Autodesk Fusion 360 part; units mm, degrees
(part 2 of 2)
sketch "Sketch4" plane through (0, 0, 5) normal (0, 0, 1) x (-1, 0, 0)
  circle A0 centre (-30, 34) radius 1.15
  circle A1 centre (-30, 82) radius 1.4
  circle A2 centre (27, 86) radius 1.15
  circle A3 centre (35, 78) radius 1.15
  circle A4 centre (31, 34) radius 1.4
  circle A5 centre (-81, 66.5) radius 1.15
  circle A6 centre (-89, 26.5) radius 1.15
  circle A7 centre (-45, 26.5) radius 1.4
  circle A8 centre (-45, 8) radius 1.15
  circle A9 centre (46, 26.5) radius 1.15
  circle A10 centre (90.029, 26.5184) radius 1.4
  circle A11 centre (90, 8) radius 1.15
  circle A12 centre (-85, 16) radius 1.15
  circle A13 centre (-85.0037, -28) radius 1.4
  circle A14 centre (-45, -32) radius 1.15
  circle A15 centre (50, -24) radius 1.15
  circle A16 centre (49.9963, -28) radius 1.4
  circle A17 centre (50, 16) radius 1.15
  circle A18 centre (-85, -32) radius 1.15
  circle A19 centre (-85, 12) radius 1.4
  circle A20 centre (90, -24) radius 1.15
  circle A21 centre (94.029, 26.5184) radius 1.15
  circle A22 centre (50, 26.5) radius 1.4
  circle A23 centre (94, 66.5) radius 1.15
  circle A24 centre (-41, 26.5) radius 1.15
  circle A25 centre (-85, 26.5) radius 1.4
  circle A26 centre (-85, 56) radius 1.15
  circle A27 centre (35, 34) radius 1.15
  circle A28 centre (35, 42) radius 1.15
  circle A29 centre (31, 86) radius 1.4
  circle A30 centre (-30, 86) radius 1.15
  circle A31 centre (-26, 34) radius 1.4
  circle A32 centre (-30, 38) radius 1.4
  circle A33 centre (-30, 78) radius 1.15
  circle A34 centre (-22, 86) radius 1.15
  circle A35 centre (35, 82) radius 1.4
  circle A36 centre (27, 34) radius 1.15
  circle A37 centre (-85, 66.5) radius 1.4
  circle A38 centre (-85, 48) radius 1.15
  circle A39 centre (-49, 26.5) radius 1.15
  circle A40 centre (-45, 12) radius 1.4
  circle A41 centre (86, 66.5) radius 1.15
  circle A42 centre (86.029, 26.5184) radius 1.15
  circle A43 centre (90, 12) radius 1.4
  circle A44 centre (90, -32) radius 1.15
  circle A45 centre (-85, -24) radius 1.15
  circle A46 centre (-45.0037, -28) radius 1.4
  circle A47 centre (50, 8) radius 1.15
  circle A48 centre (50, -32) radius 1.15
  circle A49 centre (50, 12) radius 1.4
  circle A50 centre (-45, -24) radius 1.15
  circle A51 centre (-85, 8) radius 1.15
  circle A52 centre (89.9963, -28) radius 1.4
  circle A53 centre (90, 16) radius 1.15
  circle A54 centre (54, 26.5) radius 1.15
  circle A55 centre (90, 66.5) radius 1.4
  circle A56 centre (-45, 16) radius 1.15
  circle A57 centre (-81, 26.5) radius 1.15
  circle A58 centre (-85, 52) radius 1.4
  circle A59 centre (-89, 66.5) radius 1.15
  circle A60 centre (35, 38) radius 1.4
  circle A61 centre (35, 86) radius 1.15
  circle A62 centre (-26, 86) radius 1.4
  circle A63 centre (-22, 34) radius 1.15
  circle A64 centre (-30, 42) radius 1.15
  circle A65 centre (65.5, 46) radius 2
  arc A66 (-39.1, -77.6) -> (-39.1, -74.4) centre (-39.1, -76) ccw
  line L0 (-39.1, -77.6) -> (-46.9, -77.6)
  arc A67 (-46.9, -74.4) -> (-46.9, -77.6) centre (-46.9, -76) ccw
  line L1 (-46.9, -74.4) -> (-39.1, -74.4)
  circle A68 centre (75.5, -43.5) radius 1.35
  arc A69 (-53.1, -93.6) -> (-53.1, -90.4) centre (-53.1, -92) ccw
  line L2 (-53.1, -93.6) -> (-60.9, -93.6)
  arc A70 (-60.9, -90.4) -> (-60.9, -93.6) centre (-60.9, -92) ccw
  line L3 (-60.9, -90.4) -> (-53.1, -90.4)
  arc A71 (65.9, -93.6) -> (65.9, -90.4) centre (65.9, -92) ccw
  line L4 (65.9, -93.6) -> (58.1, -93.6)
  arc A72 (58.1, -90.4) -> (58.1, -93.6) centre (58.1, -92) ccw
  line L5 (58.1, -90.4) -> (65.9, -90.4)
  circle A73 centre (-62.5, -48.623) radius 1.15
  arc A74 (51.9, -77.6) -> (51.9, -74.4) centre (51.9, -76) ccw
  line L6 (51.9, -77.6) -> (44.1, -77.6)
  arc A75 (44.1, -74.4) -> (44.1, -77.6) centre (44.1, -76) ccw
  line L7 (44.1, -74.4) -> (51.9, -74.4)
  arc A76 (90.4506, 78.0996) -> (95.5506, 78.099) centre (93.0006, 78.099) ccw
  line L8 (90.4506, 78.0996) -> (90.4506, 84.449)
  line L9 (90.4506, 84.449) -> (84.1006, 84.449)
  arc A77 (84.1006, 89.549) -> (84.1006, 84.449) centre (84.1006, 86.999) ccw
  line L10 (84.1006, 89.549) -> (92.9866, 89.549)
  arc A78 (94.8063, 88.7996) -> (92.9866, 89.549) centre (93.0006, 86.9991) ccw
  arc A79 (95.5506, 86.985) -> (94.8063, 88.7996) centre (93.0006, 86.999) ccw
  line L11 (95.5506, 86.985) -> (95.5506, 78.099)
  circle A80 centre (67.5, -48.623) radius 1.15
  arc A81 (51.9, -93.6) -> (51.9, -90.4) centre (51.9, -92) ccw
  line L12 (51.9, -93.6) -> (44.1, -93.6)
  arc A82 (44.1, -90.4) -> (44.1, -93.6) centre (44.1, -92) ccw
  line L13 (44.1, -90.4) -> (51.9, -90.4)
  arc A83 (65.9, -77.6) -> (65.9, -74.4) centre (65.9, -76) ccw
  line L14 (65.9, -77.6) -> (58.1, -77.6)
  arc A84 (58.1, -74.4) -> (58.1, -77.6) centre (58.1, -76) ccw
  line L15 (58.1, -74.4) -> (65.9, -74.4)
  circle A85 centre (-60.5, 85) radius 2
  arc A86 (-23, -94.551) -> (-22.9994, -89.451) centre (-22.9994, -92.001) ccw
  line L16 (-23, -94.551) -> (-31.8994, -94.551)
  arc A87 (-31.8994, -89.451) -> (-31.8994, -94.551) centre (-31.8994, -92.001) ccw
  line L17 (-31.8994, -89.451) -> (-22.9994, -89.451)
  circle A88 centre (-81.5, -43.5) radius 1.35
  circle A89 centre (65.5, 85) radius 2
  circle A90 centre (65.5, 65.5) radius 15
  arc A91 (36.9, -94.551) -> (36.9006, -89.451) centre (36.9006, -92.001) ccw
  line L18 (36.9, -94.551) -> (28.0006, -94.551)
  arc A92 (28.0006, -89.451) -> (28.0006, -94.551) centre (28.0006, -92.001) ccw
  line L19 (28.0006, -89.451) -> (36.9006, -89.451)
  arc A93 (-79, 84.449) -> (-78.9994, 89.549) centre (-78.9994, 86.999) ccw
  line L20 (-79, 84.449) -> (-85.3494, 84.449)
  line L21 (-85.3494, 84.449) -> (-85.3494, 78.099)
  arc A94 (-90.4494, 78.099) -> (-85.3494, 78.099) centre (-87.8994, 78.099) ccw
  line L22 (-90.4494, 78.099) -> (-90.4494, 86.9852)
  arc A95 (-89.7213, 88.7832) -> (-90.4494, 86.9852) centre (-87.8994, 86.999) ccw
  arc A96 (-87.8854, 89.549) -> (-89.7213, 88.7832) centre (-87.8994, 86.9991) ccw
  line L23 (-87.8854, 89.549) -> (-78.9994, 89.549)
  arc A97 (37.9, -77.6) -> (37.9, -74.4) centre (37.9, -76) ccw
  line L24 (37.9, -77.6) -> (30.1, -77.6)
  arc A98 (30.1, -74.4) -> (30.1, -77.6) centre (30.1, -76) ccw
  line L25 (30.1, -74.4) -> (37.9, -74.4)
  circle A99 centre (-60.5, 65.5) radius 15
  circle A100 centre (67.5, -59.5) radius 1.15
  circle A101 centre (-70.5, -43.5) radius 1.35
  arc A102 (-53.1, -77.6) -> (-53.1, -74.4) centre (-53.1, -76) ccw
  line L26 (-53.1, -77.6) -> (-60.9, -77.6)
  arc A103 (-60.9, -74.4) -> (-60.9, -77.6) centre (-60.9, -76) ccw
  line L27 (-60.9, -74.4) -> (-53.1, -74.4)
  circle A104 centre (-92.5, -43.5) radius 1.35
  arc A105 (-25.1, -77.6) -> (-25.1, -74.4) centre (-25.1, -76) ccw
  line L28 (-25.1, -77.6) -> (-32.9, -77.6)
  arc A106 (-32.9, -74.4) -> (-32.9, -77.6) centre (-32.9, -76) ccw
  line L29 (-32.9, -74.4) -> (-25.1, -74.4)
  circle A107 centre (86.5, -43.5) radius 1.35
  circle A108 centre (-62.5, -59.5) radius 1.15
  circle A109 centre (-60.5, 46) radius 2
  circle A110 centre (97.5, -43.5) radius 1.35
  arc A111 (-39.1, -93.6) -> (-39.1, -90.4) centre (-39.1, -92) ccw
  line L30 (-39.1, -93.6) -> (-46.9, -93.6)
  arc A112 (-46.9, -90.4) -> (-46.9, -93.6) centre (-46.9, -92) ccw
  line L31 (-46.9, -90.4) -> (-39.1, -90.4)
  line L32 (-67.5, -102.5) -> (72.5, -102.5)
  line L33 (72.5, -102.5) -> (72.5, -47.5)
  line L34 (72.5, -47.5) -> (102.5, -47.5)
  line L35 (102.5, -47.5) -> (102.5, 97.5)
  line L36 (102.5, 97.5) -> (-97.5, 97.5)
  line L37 (-97.5, 97.5) -> (-97.5, -47.5)
  line L38 (-97.5, -47.5) -> (-67.5, -47.5)
  line L39 (-67.5, -47.5) -> (-67.5, -102.5)
  circle A113 centre (2.5, 10) radius 1.15
  circle A114 centre (2.5, 2) radius 1.15
  circle A115 centre (-26.5, -23) radius 1.4
  circle A116 centre (23.5, -19) radius 1.15
  circle A117 centre (31.5, -19) radius 1.15
  circle A118 centre (2.5, -44) radius 1.4
  circle A119 centre (6.5, -48) radius 1.4
  circle A120 centre (10.5, -48) radius 1.15
  circle A121 centre (-5.5, -48) radius 1.15
  circle A122 centre (31.5, -23) radius 1.4
  circle A123 centre (27.5, -19) radius 1.4
  circle A124 centre (-26.5, -19) radius 1.15
  circle A125 centre (-26.5, -11) radius 1.15
  circle A126 centre (10.5, 10) radius 1.15
  circle A127 centre (-1.5, 10) radius 1.4
  circle A128 centre (2.5, 6) radius 1.4
  circle A129 centre (-26.5, -27) radius 1.15
  circle A130 centre (-18.5, -19) radius 1.15
  circle A131 centre (31.5, -15) radius 1.4
  circle A132 centre (2.5, -40) radius 1.15
  circle A133 centre (2.5, -48) radius 1.15
  circle A134 centre (-1.5, -48) radius 1.4
  circle A135 centre (31.5, -27) radius 1.15
  circle A136 centre (31.5, -11) radius 1.15
  circle A137 centre (-22.5, -19) radius 1.4
  circle A138 centre (-26.5, -15) radius 1.4
  circle A139 centre (6.5, 10) radius 1.4
  circle A140 centre (-5.5, 10) radius 1.15
  circle A141 centre (62.5, -100) radius 1.15
  circle A142 centre (-27.5, -100) radius 1.15
  circle A143 centre (47.5, -100) radius 1.15
  circle A144 centre (-57.5, -100) radius 1.15
  circle A145 centre (-42.5, -100) radius 1.15
  circle A146 centre (32.5, -100) radius 1.15
sketch "Sketch5" plane through (0, 0, 8) normal (0, 0, 1) x (-1, 0, 0)
  circle A0 centre (90.029, 26.5184) radius 1.4
  circle A1 centre (-45, 12) radius 1.4
  circle A2 centre (86, 66.5) radius 1.15
  circle A3 centre (-45, -32) radius 1.15
  circle A4 centre (50, -32) radius 1.15
  circle A5 centre (90, 66.5) radius 1.4
  circle A6 centre (-89, 26.5) radius 1.15
  circle A7 centre (-45.0037, -28) radius 1.4
  line L0 (-42, 23.5) -> (47, 23.5)
  line L1 (47, 23.5) -> (47, 15.996)
  line L2 (47, 15.996) -> (47.0104, 8.2491)
  arc A8 (47.0104, 8.2491) -> (47, 7.9983) centre (50, 8) ccw
  line L3 (47, 7.9983) -> (47, -24.0028)
  line L4 (47, -24.0028) -> (47.0072, -31.7917)
  arc A9 (47.0072, -31.7917) -> (47, -31.9983) centre (50, -32) ccw
  line L5 (47, -31.9983) -> (47, -61.5)
  line L6 (47, -61.5) -> (-42, -61.5)
  line L7 (-42, -61.5) -> (-42, 23.5)
  circle A10 centre (54, 26.5) radius 1.15
  circle A11 centre (49.9963, -28) radius 1.4
  circle A12 centre (-45, 8) radius 1.15
  circle A13 centre (-45, 16) radius 1.15
  circle A14 centre (-85, 66.5) radius 1.4
  circle A15 centre (-45, -24) radius 1.15
  circle A16 centre (50, -24) radius 1.15
  circle A17 centre (50, 16) radius 1.15
  circle A18 centre (50, 12) radius 1.4
  circle A19 centre (-81, 66.5) radius 1.15
  circle A20 centre (86.029, 26.5184) radius 1.15
  circle A21 centre (50, 26.5) radius 1.4
  circle A22 centre (50, 8) radius 1.15
  circle A23 centre (46, 26.5) radius 1.15
  circle A24 centre (-45, 26.5) radius 1.4
  circle A25 centre (-81, 26.5) radius 1.15
  circle A26 centre (94.029, 26.5184) radius 1.15
  circle A27 centre (-49, 26.5) radius 1.15
  circle A28 centre (-41, 26.5) radius 1.15
  circle A29 centre (-85, 26.5) radius 1.4
  circle A30 centre (-89, 66.5) radius 1.15
  circle A31 centre (94, 66.5) radius 1.15
  line L8 (-92.5, -40.1151) -> (-89.5, -40.1151)
  line L9 (-89.5, -40.1151) -> (-89.5, 23.542)
  arc A32 (-89.5, 23.542) -> (-88.996, 23.5) centre (-89, 26.5) ccw
  line L10 (-88.996, 23.5) -> (-81.2491, 23.5104)
  arc A33 (-81.2491, 23.5104) -> (-81.0018, 23.5) centre (-81, 26.5) ccw
  line L11 (-81.0018, 23.5) -> (-48, 23.5)
  line L12 (-48, 23.5) -> (-48, 15.996)
  line L13 (-48, 15.996) -> (-47.9896, 8.2491)
  arc A34 (-47.9896, 8.2491) -> (-48, 7.9983) centre (-45, 8) ccw
  line L14 (-48, 7.9983) -> (-48, -24.0028)
  line L15 (-48, -24.0028) -> (-47.9928, -31.7917)
  arc A35 (-47.9928, -31.7917) -> (-48, -32.0017) centre (-45, -32) ccw
  line L16 (-48, -32.0017) -> (-48, -61.5)
  line L17 (-48, -61.5) -> (-59, -61.5)
  line L18 (-59, -61.5) -> (-59, -67.5)
  line L19 (-59, -67.5) -> (-67.5, -67.5)
  line L20 (-67.5, -67.5) -> (-67.5, -70.5)
  line L21 (-67.5, -70.5) -> (-17.5, -70.5)
  line L22 (-17.5, -70.5) -> (-17.5, -97.5)
  line L23 (-17.5, -97.5) -> (-67.5, -97.5)
  line L24 (-67.5, -97.5) -> (-67.5, -102.5)
  line L25 (-67.5, -102.5) -> (-15, -102.5)
  line L26 (-15, -102.5) -> (-15, -67.5)
  line L27 (-15, -67.5) -> (20, -67.5)
  line L28 (20, -67.5) -> (20, -102.5)
  line L29 (20, -102.5) -> (72.5, -102.5)
  line L30 (72.5, -102.5) -> (72.5, -97.5)
  line L31 (72.5, -97.5) -> (22.5, -97.5)
  line L32 (22.5, -97.5) -> (22.5, -70.5)
  line L33 (22.5, -70.5) -> (72.5, -70.5)
  line L34 (72.5, -70.5) -> (72.5, -67.5)
  line L35 (72.5, -67.5) -> (64, -67.5)
  line L36 (64, -67.5) -> (64, -61.5)
  line L37 (64, -61.5) -> (53, -61.5)
  line L38 (53, -61.5) -> (53, 23.5)
  line L39 (53, 23.5) -> (94.5, 23.5)
  line L40 (94.5, 23.5) -> (94.5, -40.1151)
  line L41 (94.5, -40.1151) -> (97.5, -40.1151)
  line L42 (97.5, -40.1151) -> (97.5, 69.5047)
  line L43 (97.5, 69.5047) -> (86.2491, 69.4896)
  arc A36 (86.2491, 69.4896) -> (86, 63.5) centre (86, 66.5) ccw
  line L44 (86, 63.5) -> (94, 63.5)
  line L45 (94, 63.5) -> (94.5, 63.5)
  line L46 (94.5, 63.5) -> (94.5, 29.4812)
  arc A37 (94.5, 29.4812) -> (94.361, 29.5) centre (94.029, 26.5184) ccw
  line L47 (94.361, 29.5) -> (59, 29.5)
  line L48 (59, 29.5) -> (47, 41.5)
  line L49 (47, 41.5) -> (47, 91.5)
  line L50 (47, 91.5) -> (41, 91.5)
  line L51 (41, 91.5) -> (41, 29.5)
  line L52 (41, 29.5) -> (-36, 29.5)
  line L53 (-36, 29.5) -> (-36, 91.5)
  line L54 (-36, 91.5) -> (-42, 91.5)
  line L55 (-42, 91.5) -> (-42, 41.5)
  line L56 (-42, 41.5) -> (-54, 29.5)
  line L57 (-54, 29.5) -> (-89, 29.5)
  arc A38 (-89, 29.5) -> (-89.5, 29.458) centre (-89, 26.5) ccw
  line L58 (-89.5, 29.458) -> (-89.5, 63.5)
  line L59 (-89.5, 63.5) -> (-89, 63.5)
  line L60 (-89, 63.5) -> (-81, 63.5)
  arc A39 (-81, 63.5) -> (-81.004, 69.5) centre (-81, 66.5) ccw
  line L61 (-81.004, 69.5) -> (-88.7509, 69.4896)
  arc A40 (-88.7509, 69.4896) -> (-89.2523, 69.4894) centre (-89, 66.5) ccw
  line L62 (-89.2523, 69.4894) -> (-92.5, 69.4894)
  line L63 (-92.5, 69.4894) -> (-92.5, -40.1151)
  circle A41 centre (-57.5, -100) radius 1.15
  circle A42 centre (-57.5, -100) radius 1.15
  circle A43 centre (-42.5, -100) radius 1.15
  circle A44 centre (-27.5, -100) radius 1.15
  circle A45 centre (32.5, -100) radius 1.15
  circle A46 centre (47.5, -100) radius 1.15
  circle A47 centre (62.5, -100) radius 1.15
extrude "Extrude7" cut sketch "Sketch2" against normal blind 5 contours A209 | A210 | A211 | A212 | A213 | A214 | A215 | A216 | A217 | A218 | A219 | A220 | A221 A222 | A223 | A224 | A225 | A226 | A227 | A228 | A229 | A230 | A289 | A290 | A291 | A292 bodies 1
extrude "Extrude9" cut sketch "Sketch5" against normal blind 3 contours A41 A42 | A43 | A44 | A45 | A46 | A47 bodies 2
